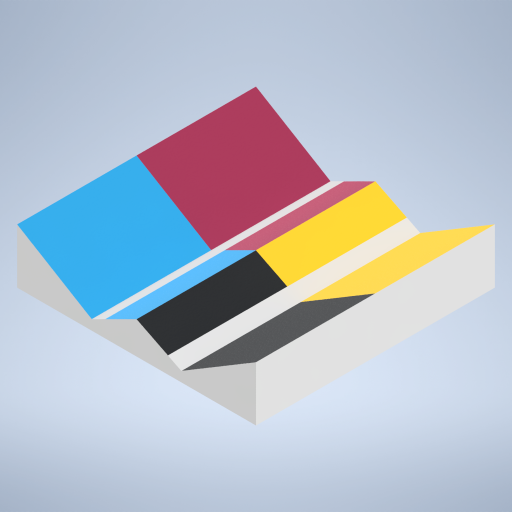
# Autodesk Inventor part: Drone Charging Base
Saved by Autodesk Inventor 2023 (Build 270158000, 158)
## iProperties
Created: 2022-12-15
Part Number: Drone Charging Base
Material: Aluminum 6061
Document SubType Name: Modeling
Designer: chase
Density: 2.7 g/cm^3
Appearance: Wall Paint: White Custom
Author: chase
Autodesk Inventor part; units mm, degrees
ref_plane "YZ Plane" through (0, 0, 0) normal (1, 0, 0) x (0, 1, 0)
ref_plane "XZ Plane" through (0, 0, 0) normal (0, 1, 0) x (-1, 0, 0)
ref_plane "XY Plane" through (0, 0, 0) normal (0, 0, 1) x (1, 0, 0)
sketch "Sketch1" plane through (0, 0, 0) normal (0, 0, 1) x (1, 0, 0)
  line L0 (0, 0) -> (1219.2, 0)
  line L1 (1219.2, 0) -> (1219.2, 279.4)
  line L2 (0, 279.4) -> (0, 0)
  line L3 (381, 50.8) -> (0, 279.4)
  line L4 (838.2, 50.8) -> (1219.2, 279.4)
  line L5 (330.2, 152.0857) -> (330.5143, 152.4)
  line L6 (787.7143, 152.4) -> (787.4, 152.4)
  line L7 (127, 152.4) -> (126.6857, 152.4)
  line L8 (381, 50.8) -> (609.6, 165.1)
  line L9 (838.2, 50.8) -> (609.6, 165.1)
  dimension "d37" = 165.1
  dimension "d39" = 457.2
  dimension "d40" = 1219.2
  dimension "d41" = 381
  dimension "d43" = 279.4
  dimension "d44" = 279.4
  dimension "d45" = 50.8
  dimension "d46" = 50.8
  dimension "d47" = 228.6
  constraints: 20 end point, 3 parallel, 1 horizontal, 1 perpendicular
  measures "d37" distance from line of L0 L8.end
  measures "d39" distance of L4.start L3.start
  measures "d40" distance of L0.start L0.end
  measures "d41" distance from line of L2 L3.start
  measures "d43" distance of L2.start L0.start
  measures "d44" distance of L0.end L1.end
  measures "d45" distance from line of L0 L3.start
  measures "d46" distance from line of L0 L4.start
  measures "d47" horizontal distance of L4.start L8.end
extrude "Extrusion3" add sketch "Sketch1" against normal blind 1219.2
sketch "Sketch3" plane through (609.6, 165.1, 0) normal (-0.4472, 0.8944, 0) x (0.8944, 0.4472, 0)
  line L0 (-179.3826, 609.6) -> (0, 609.6)
  line L1 (0, 0) -> (0, 1219.2) projected
  line L2 (-255.5826, 1219.2) -> (0, 1219.2) projected
  line L3 (-179.3826, 1219.2) -> (-179.3826, 0)
  line L4 (-255.5826, 0) -> (-255.5826, 1219.2) projected
  point P0 (-619.0778, 0)
  dimension "d52" = 76.2
  dimension "d53" = 609.6
  constraints: 4 end point, 2 perpendicular, 1 midpoint, 1 point on line
  measures "d52" distance between parallel lines of L4 L3
  measures "d53" distance from line of L3.end L0
sketch "Sketch4" plane through (838.2, 50.8, 0) normal (0.4472, 0.8944, 0) x (0.8944, -0.4472, 0)
  line L0 (0, 1219.2) -> (238.5437, 1219.2) projected
  line L1 (-76.2, 609.6) -> (-255.5826, 609.6)
  line L2 (-255.5826, 0) -> (-255.5826, 1219.2) projected
  line L3 (0, 0) -> (-255.5826, 0) projected
  line L4 (-76.2, 0) -> (-76.2, 1219.2)
  line L5 (-255.5826, 1219.2) -> (0, 1219.2) projected
  line L6 (0, 0) -> (0, 1219.2) projected
  point P0 (-726.9904, 0)
  dimension "d54" = 76.2
  constraints: 4 end point, 2 point on line, 1 midpoint, 1 perpendicular, 1 vertical
  measures "d54" distance between parallel lines of L6 L4
sketch "Sketch5" plane through (1219.2, 279.4, 0) normal (-0.5145, 0.8575, 0) x (0.8575, 0.5145, 0)
  line L0 (0, 0) -> (0, 1219.2) projected
  line L1 (0, 609.6) -> (-444.3185, 609.6)
  line L2 (-444.3185, 0) -> (-444.3185, 1219.2) projected
  point P0 (-1189.2055, 0)
  constraints: 2 end point, 2 midpoint
sketch "Sketch6" plane through (381, 50.8, 0) normal (0.5145, 0.8575, 0) x (0.8575, -0.5145, 0)
  line L0 (-444.3185, 0) -> (-444.3185, 1219.2) projected
  line L1 (-444.3185, 609.6) -> (0, 609.6)
  line L2 (0, 0) -> (0, 1219.2) projected
  point P0 (-300.5684, 0)
  constraints: 2 end point, 2 midpoint
split_face "Split1"
split_face "Split2"
split_face "Split3"
split_face "Split4"
split_face "Split5"
split_face "Split6"
body "Solid2"
